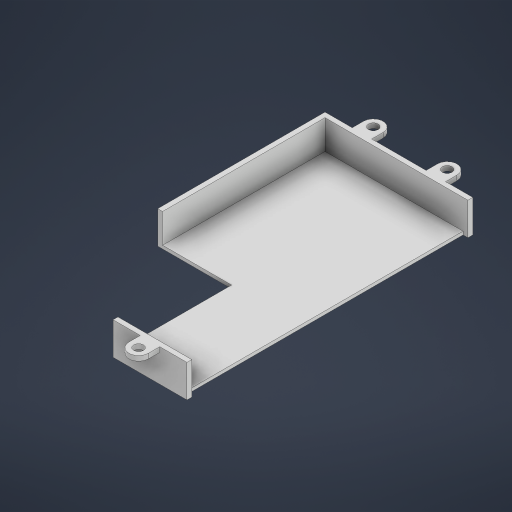
# Autodesk Inventor part: holder
Saved by Autodesk Inventor 2024.3 (Build 283343000, 343)
## iProperties
Created: 2025-08-06
Part Number: holder
Material: Generic
Document SubType Name: Modeling
Designer: giuseppe
Density: 1 g/cm^3
Appearance: Default
Author: giuseppe
Autodesk Inventor part; units mm, degrees
ref_plane "YZ Plane" through (0, 0, 0) normal (1, 0, 0) x (0, 1, 0)
ref_plane "XZ Plane" through (0, 0, 0) normal (0, 1, 0) x (-1, 0, 0)
ref_plane "XY Plane" through (0, 0, 0) normal (0, 0, 1) x (1, 0, 0)
sketch "Sketch1" plane through (0, 0, 0) normal (0, 1, 0) x (-1, 0, 0)
  line L0 (42.5, 85) -> (-42.5, 85)
  line L1 (-42.5, 85) -> (-42.5, -85)
  line L2 (-42.5, -85) -> (42.5, -85)
  line L3 (42.5, -85) -> (42.5, 85)
  line L4 (42.5, 85) -> (0, 85)
  line L5 (0, 85) -> (0, 15)
  line L6 (0, 15) -> (42.5, 15)
  line L7 (42.5, 15) -> (42.5, 85)
  point P0 (0, 0)
  point P1 (42.5, 0)
  dimension "d0" = 170
  dimension "d1" = 85
  dimension "d2" = 42.5
  dimension "d3" = 70
  constraints: 16 end point, 4 parallel, 2 horizontal, 2 midpoint, 2 perpendicular, 1 horizontal alignment, 1 vertical alignment
  measures "d0" distance of L2.end L0.start
  measures "d1" distance of L0.start L0.end
  measures "d2" distance of L5.end L6.end
  measures "d3" distance of L4.end L5.end
extrude "Extrusion1" add sketch "Sketch1" along normal blind 2 contours L5 L6 L3 L2 L1 L0
sketch "Sketch2" plane through (0, 0, 0) normal (0, -1, 0) x (1, 0, 0)
  line L0 (-42.5, -85) -> (-42.5, 15) projected
  line L1 (42.5, -85) -> (-42.5, -85) projected
  line L2 (42.5, 85) -> (42.5, -85) projected
  line L3 (0, 85) -> (42.5, 85) projected
  line L4 (0, 15) -> (0, 85) projected
  line L5 (-42.5, 15) -> (0, 15) projected
  line L6 (45.5, -88) -> (-45.5, -88)
  line L7 (-45.5, -88) -> (-45.5, 18)
  line L8 (-45.5, 18) -> (-3, 18)
  line L9 (-3, 18) -> (-3, 88)
  line L10 (-3, 88) -> (45.5, 88)
  line L11 (45.5, 88) -> (45.5, -88)
  line L12 (0, 85) -> (0, 88)
  line L13 (-42.5, 15) -> (-45.5, 15)
  line L14 (42.5, 85) -> (45.5, 85)
  line L15 (42.5, -85) -> (45.5, -85)
  point P0 (0, 0)
  dimension "d6" = 3
  constraints: 20 end point, 4 perpendicular, 4 point on line, 5 other
  measures "d6" distance between parallel lines of L2 L11
extrude "Extrusion2" add sketch "Sketch2" against normal blind 20 contours L1 L15 L11 L6 L7 L13 L0 | L3 L12 L10 L11 L14
sketch "Sketch3" plane through (0, 20, 0) normal (0, 1, 0) x (1, 0, 0)
  line L0 (16.75, -95) -> (28.75, -95)
  line L1 (28.75, -95) -> (28.75, -88)
  line L2 (28.75, -88) -> (16.75, -88)
  line L3 (16.75, -88) -> (16.75, -95)
  arc A0 (16.75, -95) -> (28.75, -95) centre (22.75, -95) ccw
  circle A1 centre (22.75, -95) radius 3
  line L4 (0, -88) -> (45.5, -88) projected
  point P0 (0, 0)
  point P1 (22.75, -88)
  point P2 (22.75, -88)
  dimension "d9" = 6
  dimension "d10" = 3
  dimension "d11" = 7
  constraints: 8 end point, 3 midpoint, 2 centre point, 2 coincident, 2 parallel, 2 point on circle, 1 collinear, 1 horizontal, 1 perpendicular
  measures "d9" diameter of A1
  measures "d10" radial gap between concentric circles of A1 A0
  measures "d11" distance of L2.end L0.start
extrude "Extrusion3" add sketch "Sketch3" against normal blind 3 contours A1 L0 L3 L2 L1 | L0 A0 A1
mirror "Mirror1" about plane through (0, 0, 0) normal (0, 0, 1) of "Extrusion3"
mirror "Mirror2" about plane through (0, 0, 0) normal (1, 0, 0) of "Extrusion3", "Mirror1"
sketch "Sketch4" plane through (-22.75, 20, 95) normal (0, 1, 0) x (1, 0, 0)
  line L0 (-17.465, -25.1497) -> (16.6088, -25.1497)
  line L1 (16.6088, -25.1497) -> (16.6088, 21.6027)
  line L2 (16.6088, 21.6027) -> (-17.465, 21.6027)
  line L3 (-17.465, 21.6027) -> (-17.465, -25.1497)
  point P0 (22.75, 95)
  constraints: 8 end point, 2 parallel, 1 horizontal, 1 perpendicular
extrude "Extrusion4" cut sketch "Sketch4" against normal blind 12.5
body "Solid1"
